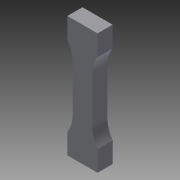
# Autodesk Inventor part: Generic DogBone
Saved by Autodesk Inventor 2014 SP1 (Build 180222100, 222)
## iProperties
Created: 2015-01-22
Part Number: Generic DogBone
Material: Generic
Document SubType Name: Modeling
Designer: Nick
Density: 1 g/cm^3
Appearance: Default
Author: Nick
Autodesk Inventor part; units mm, degrees
ref_plane "YZ Plane" through (0, 0, 0) normal (1, 0, 0) x (0, 1, 0)
ref_plane "XZ Plane" through (0, 0, 0) normal (0, 1, 0) x (-1, 0, 0)
ref_plane "XY Plane" through (0, 0, 0) normal (0, 0, 1) x (1, 0, 0)
sketch "Sketch1" plane through (0, 0, 0) normal (0, 1, 0) x (-1, 0, 0)
  line L0 (0, 0) -> (20, 0)
  line L1 (3.5, 25) -> (3.5, 40)
  line L2 (16.5, 25) -> (16.5, 40)
  arc A0 (16.5, 25) -> (20, 13.6973) centre (36.5, 25) ccw
  arc A1 (0, 13.6973) -> (3.5, 25) centre (-16.5, 25) ccw
  line L3 (3.5, 40) -> (16.5, 40) construction
  line L4 (0, 13.6973) -> (0, 0)
  line L5 (20, 13.6973) -> (20, 0)
  line L6 (0, 80) -> (20, 80)
  line L7 (3.5, 55) -> (3.5, 40)
  line L8 (16.5, 55) -> (16.5, 40)
  arc A2 (20, 66.3027) -> (16.5, 55) centre (36.5, 55) ccw
  arc A3 (3.5, 55) -> (0, 66.3027) centre (-16.5, 55) ccw
  line L9 (0, 66.3027) -> (0, 80)
  line L10 (20, 66.3027) -> (20, 80)
  dimension "d2" = 20
  dimension "d5" = 20
  dimension "d6" = 20
  dimension "d7" = 40
  dimension "d8" = 13
  dimension "d9" = 15
  constraints: 22 end point, 8 point on circle, 8 symmetric about line, 4 centre point, 2 parallel, 2 perpendicular, 2 tangent, 2 vertical alignment, 1 horizontal alignment, 1 vertical, 2 other
  measures "d2" distance of L0.start L0.end
  measures "d5" radius of A0
  measures "d6" radius of A1
  measures "d7" distance between parallel lines of L0 L3
  measures "d8" distance between parallel lines of L2 L1
  measures "d9" distance of L1.start L1.end
extrude "Extrusion1" add sketch "Sketch1" along normal blind 10
body "Solid1"
